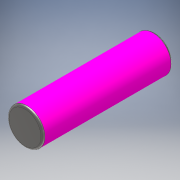
# Autodesk Inventor part: Pila_18650
Saved by Autodesk Inventor 2018.3 (Build 223285000, 285)
## iProperties
Created: 2020-11-27
Part Number: Pila_18650
Material: Acero inoxidable
Document SubType Name: Modeling
Designer: felip
Density: 8 g/cm^3
Appearance: Semipulido
Author: felip
Autodesk Inventor part; units mm, degrees
ref_plane "YZ Plane" through (0, 0, 0) normal (1, 0, 0) x (0, 1, 0)
ref_plane "XZ Plane" through (0, 0, 0) normal (0, 1, 0) x (-1, 0, 0)
ref_plane "XY Plane" through (0, 0, 0) normal (0, 0, 1) x (1, 0, 0)
sketch "Boceto1" plane through (0, 0, 0) normal (0, 1, 0) x (-1, 0, 0)
  circle A0 centre (0, 0) radius 9
  dimension "d0" = 18
  constraints: 1 centre point, 1 coincident
  measures "d0" diameter of A0
extrude "Extrusión1" add sketch "Boceto1" along normal blind 65
fillet "Empalme1" radius 1 2 edges at (9, 65, 0) (9, 0, 0)
